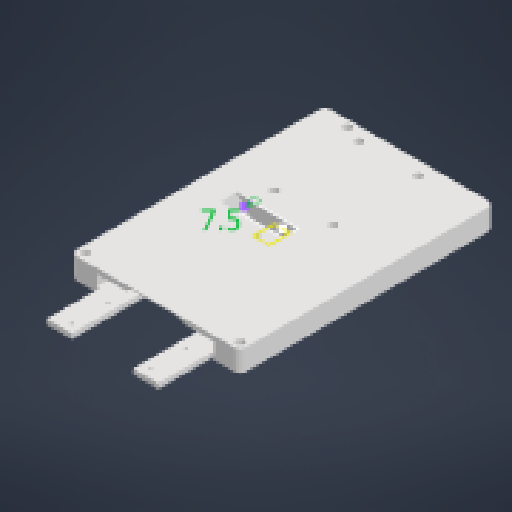
# Autodesk Inventor part: PCB_Housing_01_V4
Saved by Autodesk Inventor 2026.2 (Build 302298000, 298)
## iProperties
Created: 2026-03-15
Part Number: PCB_Housing_01_V4
Material: Generic
Document SubType Name: Modeling
Designer: vckot
Density: 1 g/cm^3
Appearance: Default
Author: vckot
Autodesk Inventor part; units mm, degrees
ref_plane "YZ Plane" through (0, 0, 0) normal (1, 0, 0) x (0, 1, 0)
ref_plane "XZ Plane" through (0, 0, 0) normal (0, 1, 0) x (-1, 0, 0)
ref_plane "XY Plane" through (0, 0, 0) normal (0, 0, 1) x (1, 0, 0)
sketch "Sketch1" plane through (0, 0, 0) normal (0, 1, 0) x (-1, 0, 0)
  line L0 (40, 60) -> (-40, 60)
  line L1 (-40, 60) -> (-40, -60)
  line L2 (-40, -60) -> (40, -60)
  line L3 (40, -60) -> (40, 60)
  line L4 (40, 60) -> (-40, -60) construction
  line L5 (-40, 60) -> (40, -60) construction
  point P0 (0, 0)
  dimension "d0" = 80
  dimension "d1" = 120
  constraints: 12 end point, 2 midpoint, 2 parallel, 1 horizontal, 1 perpendicular
  measures "d0" distance of L2.end L1.end
  measures "d1" distance of L1.end L0.end
extrude "Extrusion1" add sketch "Sketch1" along normal mid plane 10
sketch "Sketch3" plane through (0, -5, 0) normal (0, -1, 0) x (1, 0, 0)
  circle A0 centre (-36.5, 56.5) radius 2.25 projected
  circle A1 centre (36.5, 56.5) radius 2.25 projected
  circle A2 centre (-26, -56.5) radius 2.25 projected
  circle A3 centre (-17.5, -53.5) radius 2.25 projected
  circle A4 centre (10.5, -53.5) radius 2.25 projected
  circle A5 centre (-17.5, -13.5) radius 2.25 projected
  circle A6 centre (10.5, -13.5) radius 2.25 projected
  circle A7 centre (-17.5, -13.5) radius 2.25 projected
  arc A8 (8.8996, -15.0815) -> (8.8996, -11.9185) centre (10.5, -13.5) ccw projected
  point P0 (0, 0)
hole "Hole1" at (-36.5, -5, 56.5) at (36.5, -5, 56.5) at (-26, -5, -56.5) at (-17.5, -5, -53.5) at (10.5, -5, -53.5) at (-17.5, -5, -13.5) at (10.5, -5, -13.5) direction (0, 1, 0) diameter 3.75 end through all counterbore diameter 6 counterbore depth 3.5
sketch "Sketch4" plane through (40, -5, 60) normal (0, 0, 1) x (1, 0, 0)
  circle A0 centre (-40, 5) radius 4.125
  line L0 (-44.125, 0) -> (-35.875, 0)
  circle A1 centre (-50, 5) radius 2.25
  circle A2 centre (-30, 5) radius 2.25
  arc A3 (-50, 9.125) -> (-54.125, 5) centre (-50, 5) ccw
  arc A4 (-25.875, 5) -> (-30, 9.125) centre (-30, 5) ccw
  line L1 (-50, 9.125) -> (-40, 9.125)
  line L2 (-30, 9.125) -> (-40, 9.125)
  line L3 (-54.125, 5) -> (-54.125, 0)
  line L4 (-25.875, 5) -> (-25.875, 0)
  line L5 (-54.125, 0) -> (-25.875, 0)
  circle A5 centre (-40, 5) radius 2.625
  line L6 (0, 0) -> (-80, 0) projected
  point P0 (0, 10)
  point P1 (-40, 0)
  point P2 (-44.125, 0)
  dimension "d51" = 8.25
  dimension "d52" = 4.5
  dimension "d53" = 4.5
  dimension "d54" = 10
  dimension "d55" = 10
  dimension "d56" = 8.25
  dimension "d58" = 5.25
  dimension "d59" = 4.125
  dimension "d60" = 5
  dimension "d61" = 5
  constraints: 12 end point, 6 centre point, 6 point on circle, 4 coincident, 4 tangent, 2 point on line, 1 collinear, 1 horizontal, 1 midpoint, 1 perpendicular, 1 vertical alignment
  measures "d51" diameter of A0
  measures "d52" diameter of A1
  measures "d53" diameter of A2
  measures "d54" distance of A0.centre A1.centre
  measures "d55" distance of A0.centre A2.centre
  measures "d56" diameter of A3
  measures "d58" diameter of A5
  measures "d59" radius of A4
  measures "d60" vertical distance of L0.end A5.centre
  measures "d61" distance from line of A0.centre L5
extrude "Extrusion4" cut sketch "Sketch4" against normal blind 40 contours A0 | L2 A4 L4 L5 L0 L3 A3 L1 | A1 | A2 | A5
extrude "Extrusion5" cut sketch "Sketch4" against normal blind 48 contours A1 | A2
thicken "Thicken1" operation add thickness 0.25 both sides no extend neighbours yes toward (0, 1, 0) faces at (3.3333, 4.125, 46.6667) (-11.507, 3.8399, 33.3333) (-14.125, -1.6667, 33.3333) (11.2159, 3.9417, 33.3333) (14.125, -3.3333, 33.3333)
extrude "Extrusion6" cut sketch "Sketch4" against normal blind 60 contours A5
sketch "Sketch5" plane through (0, 0, 0) normal (0, 0, 1) x (1, 0, 0)
  circle A0 centre (0, 0) radius 3.75
  point P0 (0, 0)
  dimension "d63" = 7.5
  constraints: 1 centre point, 1 coincident
  measures "d63" diameter of A0
extrude "Extrusion7" cut sketch "Sketch5" along normal blind 10
sketch "Sketch6" plane through (0, 5, 0) normal (0, 1, 0) x (1, 0, 0)
  line L0 (3.75, 0) -> (3.75, -10) projected
  line L1 (-3.75, 0) -> (3.75, 0) projected
  line L2 (-3.75, 0) -> (-3.75, -10) projected
  line L3 (-3.75, -10) -> (3.75, -10) projected
  line L4 (3.75, -3.75) -> (-17.9929, -3.75)
  line L5 (-17.9929, -3.75) -> (-17.9929, 3.75)
  line L6 (-17.9929, 3.75) -> (3.75, 3.75)
  line L7 (3.75, 3.75) -> (3.75, -3.75)
  point P0 (0, 0)
  point P1 (-17.9929, 0)
  point P2 (0, 0)
  point P3 (-3.75, -3.75)
  dimension "d64" = 7.5
  constraints: 8 end point, 2 midpoint, 2 parallel, 1 horizontal, 1 horizontal alignment, 1 perpendicular, 1 point on line
  measures "d64" distance of L4.end L5.end
extrude "Extrusion8" cut sketch "Sketch6" against normal blind 7.5
sketch "Sketch7" plane through (40, -5, 60) normal (0, 0, 1) x (1, 0, 0)
  line L0 (-67.5, 2.5) -> (-12.5, 2.5)
  line L1 (-12.5, 2.5) -> (-12.5, 7.5)
  line L2 (-12.5, 7.5) -> (-67.5, 7.5)
  line L3 (-67.5, 7.5) -> (-67.5, 2.5)
  line L4 (-67.5, 2.5) -> (-12.5, 7.5) construction
  line L5 (-12.5, 2.5) -> (-67.5, 7.5) construction
  line L6 (-67.625, 2.375) -> (-12.375, 2.375)
  line L7 (-12.375, 2.375) -> (-12.375, 7.625)
  line L8 (-12.375, 7.625) -> (-67.625, 7.625)
  line L9 (-67.625, 7.625) -> (-67.625, 2.375)
  point P0 (-40, 5)
  dimension "d46" = 55
  dimension "d47" = 5
  dimension "d48" = 0.125
  constraints: 20 end point, 4 parallel, 2 midpoint, 2 perpendicular, 1 horizontal, 3 other
  measures "d46" distance of L2.end L1.end
  measures "d47" distance of L1.end L0.end
  measures "d48" distance between parallel lines of L3 L9
extrude "Extrusion9" cut sketch "Sketch7" against normal blind 36 contours L3 L2 L1 L0 | L9 L8 L7 L6
fillet "Fillet1" radius 5 1 edges at (-3.75, 1.25, 3.75)
chamfer "Chamfer2" distance 7.5 angle 45 1 edges at (-17.9929, 5, 0)
sketch "Sketch8" plane through (-40, 5, 60) normal (0, 0, 1) x (1, 0, 0)
  line L0 (25.625, -10) -> (25.625, -7.625) projected
  line L1 (25.625, -10) -> (0, -10) projected
  line L2 (25.625, -7.625) -> (13.625, -7.625)
  line L3 (13.625, -7.625) -> (13.625, -10)
  line L4 (13.625, -10) -> (25.625, -10)
  line L5 (25.625, -10) -> (25.625, -7.625)
  line L6 (54.375, -7.625) -> (66.375, -7.625)
  line L7 (66.375, -7.625) -> (66.375, -10)
  line L8 (66.375, -10) -> (54.375, -10)
  line L9 (54.375, -10) -> (54.375, -7.625)
  point P0 (40, -5)
  dimension "d71" = 12
  dimension "d72" = 12
  constraints: 16 end point, 4 parallel, 2 horizontal, 2 perpendicular, 2 point on line
  measures "d71" distance of L4.end L3.end
  measures "d72" distance of L7.end L8.end
extrude "Extrusion11" add sketch "Sketch8" along normal blind 25
sketch "Sketch9" plane through (14.375, -2.625, 24) normal (0, 1, 0) x (1, 0, 0)
  line L0 (-28.75, 0) -> (-28.75, -61) projected
  line L1 (-32.75, -57) -> (-32.75, -40) construction
  line L2 (-40.75, -36) -> (-40.75, -61) construction
  line L3 (-24.375, -36) -> (-4.375, -36) construction
  line L4 (-14.375, -36) -> (-14.375, -61) construction
  line L5 (4, -57) -> (4, -40) construction
  point P0 (-14.375, 24)
  point P1 (-32.75, -48.5)
  point P2 (-40.75, -48.5)
  point P3 (4, -48.5)
  dimension "d82" = 17
  dimension "d83" = 4
  constraints: 6 end point, 3 midpoint, 3 symmetric about line, 2 vertical, 1 horizontal alignment, 1 vertical alignment
  measures "d82" distance of L1.end L1.start
  measures "d83" distance from line of L0 L1.start
hole "Hole2" at (-18.375, -2.625, 64) at (-18.375, -2.625, 81) at (18.375, -2.625, 81) at (18.375, -2.625, 64) direction (0, -1, 0) diameter 1.5 end through all
fillet "Fillet2" radius 2 4 edges at (40, 0, 60) (40, 0, -60) (-40, 0, 60) (-40, 0, -60)
equation "\"d56\" = d51"
body "Solid1"
